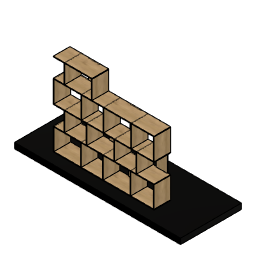
shelf v11 (Autodesk Fusion 360 design; units mm, degrees)
Autodesk Fusion 360 part; units mm, degrees
note: some values were not read from the file. Chosen so that the rebuilt part matches the saved one: which bodies a step acts on.
sketch "スケッチ1" plane through (0, 0, 0) normal (0, 1, 0) x (1, 0, 0)
  line L0 (0, 0) -> (1820, 0)
  line L1 (1820, 0) -> (1820, -300)
  line L2 (1820, -300) -> (0, -300)
  line L3 (0, -300) -> (0, 0)
  dimension "d1" = 1820
  dimension "d2" = 300
  constraint horizontal L0
  constraint vertical L1
  constraint horizontal L2
  constraint vertical L3
  constraint coincident L0.start L3.end
  measures "d1" distance of L0.start L0.end
  measures "d2" distance of L0.start L2.end
extrude "押し出し1" add sketch "スケッチ1" along normal blind 12 makes body 1
sketch "スケッチ2" plane through (0, 12, 0) normal (0, 1, 0) x (-1, 0, 0)
  line L0 (0, 300) -> (-1820, 300)
  line L1 (-1820, 300) -> (-1820, 0)
  line L2 (-1820, 0) -> (0, 0)
  line L3 (0, 0) -> (0, 300)
  line L4 (0, 0) -> (-12, 0)
  line L5 (-12, 0) -> (-12, 300)
  line L6 (-12, 300) -> (0, 300)
  line L7 (0, 300) -> (0, 0)
  line L8 (-12, 0) -> (-494, 0)
  line L9 (-494, 0) -> (-494, 300)
  line L10 (-494, 300) -> (-12, 300)
  line L11 (-12, 300) -> (-12, 0)
  line L12 (-494, 0) -> (-506, 0)
  line L13 (-506, 0) -> (-506, 300)
  line L14 (-506, 300) -> (-494, 300)
  line L15 (-494, 300) -> (-494, 0)
  line L16 (-506, 0) -> (-890, 0)
  line L17 (-890, 0) -> (-890, 300)
  line L18 (-890, 300) -> (-506, 300)
  line L19 (-506, 300) -> (-506, 0)
  line L20 (-890, 0) -> (-902, 0)
  line L21 (-902, 0) -> (-902, 300)
  line L22 (-902, 300) -> (-890, 300)
  line L23 (-890, 300) -> (-890, 0)
  line L24 (-902, 0) -> (-1290, 0)
  line L25 (-1290, 0) -> (-1290, 300)
  line L26 (-1290, 300) -> (-902, 300)
  line L27 (-902, 300) -> (-902, 0)
  dimension "d5" = 12
  dimension "d6" = 482
  dimension "d7" = 12
  dimension "d8" = 384
  dimension "d9" = 300
  dimension "d10" = 12
  dimension "d11" = 388
  constraint horizontal L4
  constraint vertical L5
  constraint horizontal L6
  constraint vertical L7
  constraint coincident L2.end L3.start
  constraint horizontal L8
  constraint vertical L9
  constraint horizontal L10
  constraint vertical L11
  constraint horizontal L12
  constraint vertical L13
  constraint horizontal L14
  constraint vertical L15
  constraint horizontal L16
  constraint vertical L17
  constraint horizontal L18
  constraint vertical L19
  constraint horizontal L20
  constraint vertical L21
  constraint horizontal L22
  constraint vertical L23
  constraint horizontal L24
  constraint vertical L25
  constraint horizontal L26
  constraint vertical L27
  measures "d5" distance of L2.end L4.end
  measures "d6" distance of L4.end L8.end
  measures "d7" distance of L8.end L12.end
  measures "d8" distance of L12.end L16.end
  measures "d9" distance of L12.end L13.end
  measures "d10" distance of L16.end L20.end
  measures "d11" distance of L20.end L24.end
sketch "スケッチ3" plane through (0, 12, 0) normal (0, 1, 0) x (-1, 0, 0)
  line L0 (-900, 0) -> (-1388, 0)
  line L1 (-1388, 0) -> (-1388, 300)
  line L2 (-1388, 300) -> (-900, 300)
  line L3 (-900, 300) -> (-900, 0)
  line L4 (-1820, 0) -> (-1808, 0)
  line L5 (-1808, 0) -> (-1808, 300)
  line L6 (-1808, 300) -> (-1820, 300)
  line L7 (-1820, 300) -> (-1820, 0)
  line L8 (-1388, 0) -> (-1808, 0)
  line L9 (-1808, 0) -> (-1808, 300)
  line L10 (-1808, 300) -> (-1388, 300)
  line L11 (-1388, 300) -> (-1388, 0)
  line L12 (-1388, 0) -> (-1400, 0)
  line L13 (-1400, 0) -> (-1400, 300)
  line L14 (-1400, 300) -> (-1388, 300)
  line L15 (-1388, 300) -> (-1388, 0)
  dimension "d12" = 488
  dimension "d13" = 12
  dimension "d14" = 300
  dimension "d15" = 12
  constraint horizontal L0
  constraint vertical L1
  constraint horizontal L2
  constraint vertical L3
  constraint horizontal L4
  constraint vertical L5
  constraint horizontal L6
  constraint vertical L7
  constraint horizontal L8
  constraint vertical L9
  constraint horizontal L10
  constraint vertical L11
  constraint horizontal L12
  constraint vertical L13
  constraint horizontal L14
  constraint vertical L15
  measures "d12" distance of L0.start L0.end
  measures "d13" distance of L4.start L4.end
  measures "d14" distance of L0.end L1.end
  measures "d15" distance of L0.end L12.end
extrude "押し出し2" add sketch "スケッチ3" sketch "スケッチ2" along normal blind 382 separate body contours L1 L8 L10 L11 L12 L13 L14 L15 | L4 L5 L6 L7 L9 of sketch 2 contours L0 L2 L3 L4 L5 L6 L7 L11 | L0 L2 L9 L12 L13 L14 L15 L19 | L0 L2 L17 L20 L21 L22 L23 L27 makes body 2 at (0, 266.6667, 100) makes body 3 at (1820, 266.6667, 200) makes body 4 at (1400, 266.6667, 100) makes body 5 at (494, 266.6667, 100) makes body 6 at (890, 266.6667, 100)
sketch "スケッチ7" plane through (0, 394, 0) normal (0, 1, 0) x (-1, 0, 0)
  line L0 (0, 300) -> (-12, 300)
  line L1 (-12, 300) -> (-12, 0)
  line L2 (-12, 0) -> (0, 0)
  line L3 (0, 0) -> (0, 300)
  line L4 (0, 0) -> (-1820, 0)
  line L5 (-1820, 0) -> (-1820, 300)
  line L6 (-1820, 300) -> (0, 300)
  line L7 (0, 300) -> (0, 0)
  constraint horizontal L4
  constraint vertical L5
  constraint horizontal L6
  constraint vertical L7
  constraint coincident L2.end L3.start
extrude "押し出し4" add sketch "スケッチ7" along normal blind 12 separate body contours L1 L4 L5 L6 makes body 7
extrude "押し出し5" add 1 faces at (12, 398, 200) along direction (-1, 0, 0) blind 12 on bodies 7 bodies 7 2
split "分割1" by plane through (0, 394, 0) normal (0, -1, 0) bodies 7 makes body 8 at (0, 139.3333, 200)
sketch "スケッチ8" plane through (0, 406, 0) normal (0, 1, 0) x (-1, 0, 0)
  line L0 (-1820, 300) -> (-1820, 0)
  line L1 (-1820, 0) -> (0, 0)
  line L2 (0, 0) -> (0, 300)
  line L3 (0, 300) -> (-1820, 300)
  line L4 (0, 0) -> (-194, 0)
  line L5 (-194, 0) -> (-194, 300)
  line L6 (-194, 300) -> (0, 300)
  line L7 (0, 300) -> (0, 0)
  line L8 (-194, 0) -> (-206, 0)
  line L9 (-206, 0) -> (-206, 300)
  line L10 (-206, 300) -> (-194, 300)
  line L11 (-194, 300) -> (-194, 0)
  line L12 (-206, 0) -> (-594, 0)
  line L13 (-594, 0) -> (-594, 300)
  line L14 (-594, 300) -> (-206, 300)
  line L15 (-206, 300) -> (-206, 0)
  line L16 (-594, 0) -> (-606, 0)
  line L17 (-606, 0) -> (-606, 300)
  line L18 (-606, 300) -> (-594, 300)
  line L19 (-594, 300) -> (-594, 0)
  line L20 (-606, 0) -> (-1094, 0)
  line L21 (-1094, 0) -> (-1094, 300)
  line L22 (-1094, 300) -> (-606, 300)
  line L23 (-606, 300) -> (-606, 0)
  line L24 (-1094, 0) -> (-1106, 0)
  line L25 (-1106, 0) -> (-1106, 300)
  line L26 (-1106, 300) -> (-1094, 300)
  line L27 (-1094, 300) -> (-1094, 0)
  line L28 (-1106, 0) -> (-1494, 0)
  line L29 (-1494, 0) -> (-1494, 300)
  line L30 (-1494, 300) -> (-1106, 300)
  line L31 (-1106, 300) -> (-1106, 0)
  line L32 (-1494, 0) -> (-1506, 0)
  line L33 (-1506, 0) -> (-1506, 300)
  line L34 (-1506, 300) -> (-1494, 300)
  line L35 (-1494, 300) -> (-1494, 0)
  dimension "d34" = 194
  dimension "d35" = 12
  dimension "d36" = 388
  dimension "d37" = 300
  dimension "d38" = 12
  dimension "d39" = 488
  dimension "d40" = 12
  dimension "d41" = 388
  dimension "d42" = 300
  dimension "d43" = 12
  constraint horizontal L4
  constraint vertical L5
  constraint horizontal L6
  constraint vertical L7
  constraint coincident L1.end L2.start
  constraint horizontal L8
  constraint vertical L9
  constraint horizontal L10
  constraint vertical L11
  constraint horizontal L12
  constraint vertical L13
  constraint horizontal L14
  constraint vertical L15
  constraint horizontal L16
  constraint vertical L17
  constraint horizontal L18
  constraint vertical L19
  constraint horizontal L20
  constraint vertical L21
  constraint horizontal L22
  constraint vertical L23
  constraint horizontal L24
  constraint vertical L25
  constraint horizontal L26
  constraint vertical L27
  constraint horizontal L28
  constraint vertical L29
  constraint horizontal L30
  constraint vertical L31
  constraint horizontal L32
  constraint vertical L33
  constraint horizontal L34
  constraint vertical L35
  measures "d34" distance of L1.end L4.end
  measures "d35" distance of L4.end L8.end
  measures "d36" distance of L8.end L12.end
  measures "d37" distance of L8.end L9.end
  measures "d38" distance of L12.end L16.end
  measures "d39" distance of L16.end L20.end
  measures "d40" distance of L20.end L24.end
  measures "d41" distance of L24.end L28.end
  measures "d42" distance of L24.end L25.end
  measures "d43" distance of L28.end L32.end
extrude "押し出し6" add sketch "スケッチ8" along normal blind 338 separate body contours L1 L3 L29 L32 L33 L34 L35 | L1 L3 L21 L24 L25 L26 L27 L31 | L1 L3 L13 L16 L17 L18 L19 L23 | L1 L3 L5 L8 L9 L10 L11 L15 makes body 9 at (594, 631.3333, 100) makes body 10 at (1094, 631.3333, 100) makes body 11 at (194, 631.3333, 100) makes body 12 at (1494, 631.3333, 100)
sketch "スケッチ9" plane through (0, 744, 0) normal (0, 1, 0) x (-1, 0, 0)
  line L0 (-194, 300) -> (-206, 300)
  line L1 (-206, 300) -> (-206, 0)
  line L2 (-206, 0) -> (-194, 0)
  line L3 (-194, 0) -> (-194, 300)
  line L4 (0, 0) -> (-1820, 0)
  line L5 (-1820, 0) -> (-1820, 300)
  line L6 (-1820, 300) -> (0, 300)
  line L7 (0, 300) -> (0, 0)
  constraint horizontal L4
  constraint vertical L5
  constraint horizontal L6
  constraint vertical L7
  constraint coincident L4.start L7.end
extrude "押し出し7" add sketch "スケッチ9" along normal blind 12 separate body contours L1 L4 L5 L6 makes body 13
move_face "面をオフセット1" offset 200 1 faces at (206, 748, 200) on bodies 13
extrude "押し出し8" add 1 faces at (6, 748, 200) along direction (-1, 0, 0) blind 6 on bodies 13 bodies 13
sketch "スケッチ10" plane through (0, 756, 0) normal (0, 1, 0) x (-1, 0, 0)
  line L0 (-1820, 300) -> (-1820, 0)
  line L1 (-1820, 0) -> (0, 0)
  line L2 (0, 0) -> (0, 300)
  line L3 (0, 300) -> (-1820, 300)
  line L4 (0, 0) -> (-12, 0)
  line L5 (-12, 0) -> (-12, 300)
  line L6 (-12, 300) -> (0, 300)
  line L7 (0, 300) -> (0, 0)
  line L8 (-12, 0) -> (-500, 0)
  line L9 (-500, 0) -> (-500, 300)
  line L10 (-500, 300) -> (-12, 300)
  line L11 (-12, 300) -> (-12, 0)
  line L12 (-500, 0) -> (-512, 0)
  line L13 (-512, 0) -> (-512, 300)
  line L14 (-512, 300) -> (-500, 300)
  line L15 (-500, 300) -> (-500, 0)
  line L16 (-512, 0) -> (-900, 0)
  line L17 (-900, 0) -> (-900, 300)
  line L18 (-900, 300) -> (-512, 300)
  line L19 (-512, 300) -> (-512, 0)
  line L20 (-900, 0) -> (-912, 0)
  line L21 (-912, 0) -> (-912, 300)
  line L22 (-912, 300) -> (-900, 300)
  line L23 (-900, 300) -> (-900, 0)
  line L24 (-912, 0) -> (-1400, 0)
  line L25 (-1400, 0) -> (-1400, 300)
  line L26 (-1400, 300) -> (-912, 300)
  line L27 (-912, 300) -> (-912, 0)
  line L28 (-1400, 0) -> (-1412, 0)
  line L29 (-1412, 0) -> (-1412, 300)
  line L30 (-1412, 300) -> (-1400, 300)
  line L31 (-1400, 300) -> (-1400, 0)
  line L32 (-1412, 0) -> (-1808, 0)
  line L33 (-1808, 0) -> (-1808, 300)
  line L34 (-1808, 300) -> (-1412, 300)
  line L35 (-1412, 300) -> (-1412, 0)
  dimension "d51" = 12
  dimension "d52" = 488
  dimension "d53" = 12
  dimension "d54" = 388
  dimension "d55" = 12
  dimension "d56" = 488
  dimension "d57" = 12
  dimension "d58" = 396
  dimension "d59" = 300
  constraint horizontal L4
  constraint vertical L5
  constraint horizontal L6
  constraint vertical L7
  constraint coincident L1.end L2.start
  constraint horizontal L8
  constraint vertical L9
  constraint horizontal L10
  constraint vertical L11
  constraint horizontal L12
  constraint vertical L13
  constraint horizontal L14
  constraint vertical L15
  constraint horizontal L16
  constraint vertical L17
  constraint horizontal L18
  constraint vertical L19
  constraint horizontal L20
  constraint vertical L21
  constraint horizontal L22
  constraint vertical L23
  constraint horizontal L24
  constraint vertical L25
  constraint horizontal L26
  constraint vertical L27
  constraint horizontal L28
  constraint vertical L29
  constraint horizontal L30
  constraint vertical L31
  constraint horizontal L32
  constraint vertical L33
  constraint horizontal L34
  constraint vertical L35
  measures "d51" distance of L1.end L4.end
  measures "d52" distance of L4.end L8.end
  measures "d53" distance of L8.end L12.end
  measures "d54" distance of L12.end L16.end
  measures "d55" distance of L16.end L20.end
  measures "d56" distance of L20.end L24.end
  measures "d57" distance of L24.end L28.end
  measures "d58" distance of L28.end L32.end
  measures "d59" distance of L28.end L29.end
extrude "押し出し9" add sketch "スケッチ10" along normal blind 388 separate body contours L0 L1 L3 L33 | L1 L3 L25 L28 L29 L30 L31 L35 | L1 L3 L17 L20 L21 L22 L23 L27 | L1 L3 L9 L12 L13 L14 L15 L19 | L1 L2 L3 L4 L5 L6 L7 L11 makes body 14 at (900, 1014.6667, 100) makes body 15 at (1400, 1014.6667, 100) makes body 16 at (500, 1014.6667, 100) makes body 17 at (1820, 1014.6667, 200) makes body 18 at (0, 1014.6667, 100)
sketch "スケッチ11" plane through (0, 1144, 0) normal (0, 1, 0) x (-1, 0, 0)
  line L0 (0, 300) -> (-12, 300)
  line L1 (-12, 300) -> (-12, 0)
  line L2 (-12, 0) -> (0, 0)
  line L3 (0, 0) -> (0, 300)
  line L4 (0, 0) -> (-1820, 0)
  line L5 (-1820, 0) -> (-1820, 300)
  line L6 (-1820, 300) -> (0, 300)
  line L7 (0, 300) -> (0, 0)
  constraint horizontal L4
  constraint vertical L5
  constraint horizontal L6
  constraint vertical L7
  constraint coincident L2.end L3.start
extrude "押し出し10" add sketch "スケッチ11" along normal blind 12 separate body makes body 19
sketch "スケッチ12" plane through (0, 1156, 0) normal (0, 1, 0) x (-1, 0, 0)
  line L0 (0, 300) -> (-1820, 300)
  line L1 (-1820, 300) -> (-1820, 0)
  line L2 (-1820, 0) -> (0, 0)
  line L3 (0, 0) -> (0, 300)
  line L4 (0, 0) -> (-12, 0)
  line L5 (-12, 0) -> (-12, 300)
  line L6 (-12, 300) -> (0, 300)
  line L7 (0, 300) -> (0, 0)
  line L8 (-12, 0) -> (-194, 0)
  line L9 (-194, 0) -> (-194, 300)
  line L10 (-194, 300) -> (-12, 300)
  line L11 (-12, 300) -> (-12, 0)
  line L12 (-194, 0) -> (-206, 0)
  line L13 (-206, 0) -> (-206, 300)
  line L14 (-206, 300) -> (-194, 300)
  line L15 (-194, 300) -> (-194, 0)
  line L16 (-206, 0) -> (-688, 0)
  line L17 (-688, 0) -> (-688, 300)
  line L18 (-688, 300) -> (-206, 300)
  line L19 (-206, 300) -> (-206, 0)
  line L20 (-688, 0) -> (-700, 0)
  line L21 (-700, 0) -> (-700, 300)
  line L22 (-700, 300) -> (-688, 300)
  line L23 (-688, 300) -> (-688, 0)
  dimension "d64" = 12
  dimension "d65" = 182
  dimension "d66" = 12
  dimension "d67" = 482
  dimension "d68" = 300
  dimension "d69" = 12
  constraint horizontal L4
  constraint vertical L5
  constraint horizontal L6
  constraint vertical L7
  constraint coincident L2.end L3.start
  constraint horizontal L8
  constraint vertical L9
  constraint horizontal L10
  constraint vertical L11
  constraint horizontal L12
  constraint vertical L13
  constraint horizontal L14
  constraint vertical L15
  constraint horizontal L16
  constraint vertical L17
  constraint horizontal L18
  constraint vertical L19
  constraint horizontal L20
  constraint vertical L21
  constraint horizontal L22
  constraint vertical L23
  measures "d64" distance of L2.end L4.end
  measures "d65" distance of L4.end L8.end
  measures "d66" distance of L8.end L12.end
  measures "d67" distance of L12.end L16.end
  measures "d68" distance of L12.end L13.end
  measures "d69" distance of L16.end L20.end
sketch "スケッチ13" plane through (0, 1488, 0) normal (0, 1, 0) x (-1, 0, 0)
  line L0 (0, 300) -> (-12, 300)
  line L1 (-12, 300) -> (-12, 0)
  line L2 (-12, 0) -> (0, 0)
  line L3 (0, 0) -> (0, 300)
  line L4 (0, 0) -> (-700, 0)
  line L5 (-700, 0) -> (-700, 300)
  line L6 (-700, 300) -> (0, 300)
  line L7 (0, 300) -> (0, 0)
  constraint horizontal L4
  constraint vertical L5
  constraint horizontal L6
  constraint vertical L7
  constraint coincident L2.end L3.start
extrude "押し出し12" add sketch "スケッチ13" along normal blind 12 separate body makes body 20
sketch "スケッチ14" plane through (0, 0, 0) normal (0, 0, -1) x (-1, 0, 0)
  line L0 (-1820, 394) -> (0, 394)
  line L1 (0, 394) -> (0, 406)
  line L2 (0, 406) -> (-1820, 406)
  line L3 (-1820, 406) -> (-1820, 394)
  line L4 (-402.3819, 406) -> (-222.3819, 406)
  line L5 (-222.3819, 406) -> (-222.3819, 0)
  line L6 (-222.3819, 0) -> (-402.3819, 0)
  line L7 (-402.3819, 0) -> (-402.3819, 406)
  dimension "d74" = 180
  constraint horizontal L4
  constraint vertical L5
  constraint horizontal L6
  constraint vertical L7
  constraint coincident L2 L4.start
  measures "d74" distance of L4.start L4.end
extrude "押し出し13" add sketch "スケッチ14" along normal blind 12 separate body contours L0 L2 L4 L5 L7 | L0 L5 L6 L7 makes body 21
sketch "スケッチ15" plane through (0, 0, 0) normal (0, 0, -1) x (-1, 0, 0)
  line L0 (-1820, 744) -> (0, 744)
  line L1 (0, 744) -> (0, 756)
  line L2 (0, 756) -> (-1820, 756)
  line L3 (-1820, 756) -> (-1820, 744)
  line L4 (-400.5318, 1143.8543) -> (-220.5318, 1143.8543)
  line L5 (-220.5318, 1143.8543) -> (-220.5318, 755.8543)
  line L6 (-220.5318, 755.8543) -> (-400.5318, 755.8543)
  line L7 (-400.5318, 755.8543) -> (-400.5318, 1143.8543)
  dimension "d77" = 180
  dimension "d78" = 388
  constraint horizontal L4
  constraint vertical L5
  constraint horizontal L6
  constraint vertical L7
  measures "d77" distance of L4.start L4.end
  measures "d78" distance of L4.start L6.end
extrude "押し出し14" add sketch "スケッチ15" along normal blind 12 separate body contours L2 L4 L5 L7 makes body 22
move_body "移動5" bodies 22 to x (1, 0, 0) y (0, 1, 0) z (0, 0, 1) at (0, 0, 12)
sketch "スケッチ16" plane through (0, 0, 0) normal (0, 0, -1) x (-1, 0, 0)
  line L0 (-700, 1488) -> (0, 1488)
  line L1 (0, 1488) -> (0, 1500)
  line L2 (0, 1500) -> (-700, 1500)
  line L3 (-700, 1500) -> (-700, 1488)
  line L4 (-548.7632, 1488) -> (-398.7632, 1488)
  line L5 (-398.7632, 1488) -> (-398.7632, 1156)
  line L6 (-398.7632, 1156) -> (-548.7632, 1156)
  line L7 (-548.7632, 1156) -> (-548.7632, 1488)
  dimension "d81" = 150
  dimension "d82" = 332
  constraint horizontal L4
  constraint vertical L5
  constraint horizontal L6
  constraint vertical L7
  constraint coincident L0 L4.start
  measures "d81" distance of L4.start L4.end
  measures "d82" distance of L4.start L6.end
extrude "押し出し15" add sketch "スケッチ16" against normal blind 12 separate body contours L0 L4 L5 L6 L7 makes body 23
move_body "移動6" bodies 23 to x (1, 0, 0) y (0, 1, 0) z (0, 0, 1) at (0, 0, -100)
extrude "押し出し16" add 1 faces at (398.7632, 1377.3333, -96) along direction (-1, 0, 0) blind 50 on bodies 23 bodies 23
move_body "移動7" bodies 23 to x (1, 0, 0) y (0, 1, 0) z (0, 0, 1) at (0, 0, 100)
sketch "スケッチ17" plane through (0, 0, 0) normal (0, 0, -1) x (-1, 0, 0)
  line L0 (-1820, 744) -> (0, 744)
  line L1 (0, 744) -> (0, 756)
  line L2 (0, 756) -> (-1820, 756)
  line L3 (-1820, 756) -> (-1820, 744)
  line L4 (-923.4026, 744) -> (-723.4026, 744)
  line L5 (-723.4026, 744) -> (-723.4026, 406)
  line L6 (-723.4026, 406) -> (-923.4026, 406)
  line L7 (-923.4026, 406) -> (-923.4026, 744)
  dimension "d87" = 200
  dimension "d88" = 338
  constraint horizontal L4
  constraint vertical L5
  constraint horizontal L6
  constraint vertical L7
  constraint coincident L0 L4.start
  measures "d87" distance of L4.start L4.end
  measures "d88" distance of L4.start L6.end
sketch "スケッチ18" plane through (0, 0, 0) normal (0, 0, -1) x (-1, 0, 0)
  line L0 (-1820, 1144) -> (0, 1144)
  line L1 (0, 1144) -> (0, 1156)
  line L2 (0, 1156) -> (-1820, 1156)
  line L3 (-1820, 1156) -> (-1820, 1144)
  line L4 (-1299.0932, 1144) -> (-1099.0932, 1144)
  line L5 (-1099.0932, 1144) -> (-1099.0932, 756)
  line L6 (-1099.0932, 756) -> (-1299.0932, 756)
  line L7 (-1299.0932, 756) -> (-1299.0932, 1144)
  dimension "d89" = 200
  dimension "d90" = 388
  constraint horizontal L4
  constraint vertical L5
  constraint horizontal L6
  constraint vertical L7
  constraint coincident L0 L4.start
  measures "d89" distance of L4.start L4.end
  measures "d90" distance of L4.start L6.end
sketch "スケッチ19" plane through (0, 0, 0) normal (0, 0, -1) x (-1, 0, 0)
  line L0 (-1820, 394) -> (0, 394)
  line L1 (0, 394) -> (0, 406)
  line L2 (0, 406) -> (-1820, 406)
  line L3 (-1820, 406) -> (-1820, 394)
  line L4 (-1271.1858, 394) -> (-1071.1858, 394)
  line L5 (-1071.1858, 394) -> (-1071.1858, 12)
  line L6 (-1071.1858, 12) -> (-1271.1858, 12)
  line L7 (-1271.1858, 12) -> (-1271.1858, 394)
  dimension "d91" = 200
  dimension "d92" = 382
  constraint horizontal L4
  constraint vertical L5
  constraint horizontal L6
  constraint vertical L7
  constraint coincident L0 L4.start
  measures "d91" distance of L4.start L4.end
  measures "d92" distance of L4.start L6.end
extrude "押し出し17" cut 1 faces at (282.3819, 0, -8) along direction (0, 1, 0) blind 24 on bodies 21 bodies 21
move_body "移動8" bodies 21 to x (1, 0, 0) y (0, 1, 0) z (0, 0, 1) at (0, -12, 12)
extrude "押し出し18" add sketch "スケッチ17" sketch "スケッチ18" sketch "スケッチ19" against normal blind 12 separate body contours L0 L4 L5 L6 L7 of sketch 2 contours L0 L4 L5 L6 L7 of sketch 3 contours L0 L4 L5 L6 L7 makes body 24 at (1165.7599, 885.3333, 0) makes body 25 at (856.7359, 631.3333, 0) makes body 26 at (1204.5191, 266.6667, 0)
sketch "スケッチ20" plane through (0, 1488, 0) normal (0, -1, 0) x (1, 0, 0)
  line L0 (700, 300) -> (0, 300)
  line L1 (0, 300) -> (0, 0)
  line L2 (0, 0) -> (700, 0)
  line L3 (700, 0) -> (700, 300)
  line L4 (700, 300) -> (688, 300)
  line L5 (688, 300) -> (688, 0)
  line L6 (688, 0) -> (700, 0)
  line L7 (700, 0) -> (700, 300)
  line L8 (688, 300) -> (206, 300)
  line L9 (206, 300) -> (206, 0)
  line L10 (206, 0) -> (688, 0)
  line L11 (688, 0) -> (688, 300)
  line L12 (206, 300) -> (194, 300)
  line L13 (194, 300) -> (194, 0)
  line L14 (194, 0) -> (206, 0)
  line L15 (206, 0) -> (206, 300)
  dimension "d97" = 12
  dimension "d98" = 482
  dimension "d99" = 12
  constraint horizontal L4
  constraint vertical L5
  constraint horizontal L6
  constraint vertical L7
  constraint coincident L0.start L3.end
  constraint horizontal L8
  constraint vertical L9
  constraint horizontal L10
  constraint vertical L11
  constraint horizontal L12
  constraint vertical L13
  constraint horizontal L14
  constraint vertical L15
  measures "d97" distance of L0.start L4.end
  measures "d98" distance of L4.end L8.end
  measures "d99" distance of L8.end L12.end
extrude "押し出し19" add sketch "スケッチ20" along normal blind 332 separate body contours L0 L2 L3 L4 L5 L6 L7 L11 | L0 L2 L9 L12 L13 L14 L15 makes body 27 at (700, 1377.3333, 100) makes body 28 at (206, 1377.3333, 200)
sketch "スケッチ21" plane through (0, 0, 0) normal (0, 1, 0) x (1, 0, 0)
  line L0 (-500, -500) -> (2500, -500)
  line L1 (2500, -500) -> (2500, 600)
  line L2 (2500, 600) -> (-500, 600)
  line L3 (-500, 600) -> (-500, -500)
  constraint horizontal L0
  constraint vertical L1
  constraint horizontal L2
  constraint vertical L3
extrude "押し出し20" add sketch "スケッチ21" against normal blind 100 separate body makes body 29
copy_body "ボディのコピーと貼り付け5" bodies 25 makes body 30
move_body "移動9" bodies 30 to x (1, 0, 0) y (0, 1, 0) z (0, 0, 1) at (850, 0, 0)
sketch "スケッチ4" plane through (0, 394, 0) normal (0, 1, 0) x (-1, 0, 0)
  line L0 (0, 0) -> (-1820, 0)
  line L1 (-1820, 0) -> (-1820, 300)
  line L2 (-1820, 300) -> (0, 300)
  line L3 (0, 300) -> (0, 0)
  line L4 (0, 0) -> (-140, 0)
  line L5 (-140, 0) -> (-140, 300)
  line L6 (-140, 300) -> (0, 300)
  line L7 (0, 300) -> (0, 0)
  line L8 (-140, 0) -> (-152, 0)
  line L9 (-152, 0) -> (-152, 300)
  line L10 (-152, 300) -> (-140, 300)
  line L11 (-140, 300) -> (-140, 0)
  line L12 (-152, 0) -> (-540, 0)
  line L13 (-540, 0) -> (-540, 300)
  line L14 (-540, 300) -> (-152, 300)
  line L15 (-152, 300) -> (-152, 0)
  line L16 (-540, 0) -> (-552, 0)
  line L17 (-552, 0) -> (-552, 300)
  line L18 (-552, 300) -> (-540, 300)
  line L19 (-540, 300) -> (-540, 0)
  line L20 (-552, 0) -> (-1040, 0)
  line L21 (-1040, 0) -> (-1040, 300)
  line L22 (-1040, 300) -> (-552, 300)
  line L23 (-552, 300) -> (-552, 0)
  line L24 (-1040, 0) -> (-1052, 0)
  line L25 (-1052, 0) -> (-1052, 300)
  line L26 (-1052, 300) -> (-1040, 300)
  line L27 (-1040, 300) -> (-1040, 0)
  line L28 (-890, 300) -> (-902, 300)
  line L29 (-902, 300) -> (-902, 0)
  line L30 (-902, 0) -> (-890, 0)
  line L31 (-890, 0) -> (-890, 300)
  line L32 (-494, 300) -> (-506, 300)
  line L33 (-506, 300) -> (-506, 0)
  line L34 (-506, 0) -> (-494, 0)
  line L35 (-494, 0) -> (-494, 300)
  line L36 (-1388, 300) -> (-1400, 300)
  line L37 (-1400, 300) -> (-1400, 0)
  line L38 (-1400, 0) -> (-1388, 0)
  line L39 (-1388, 0) -> (-1388, 300)
  line L40 (-1808, 0) -> (-1808, 300)
  line L41 (-1808, 300) -> (-1820, 300)
  line L42 (-1820, 300) -> (-1820, 0)
  line L43 (-1820, 0) -> (-1808, 0)
  dimension "d18" = 140
  dimension "d19" = 12
  dimension "d20" = 300
  dimension "d21" = 388
  dimension "d22" = 12
  dimension "d23" = 488
  dimension "d24" = 300
  dimension "d25" = 12
  constraint horizontal L0
  constraint vertical L1
  constraint horizontal L2
  constraint vertical L3
  constraint horizontal L4
  constraint vertical L5
  constraint horizontal L6
  constraint vertical L7
  constraint horizontal L8
  constraint vertical L9
  constraint horizontal L10
  constraint vertical L11
  constraint horizontal L12
  constraint vertical L13
  constraint horizontal L14
  constraint vertical L15
  constraint horizontal L16
  constraint vertical L17
  constraint horizontal L18
  constraint vertical L19
  constraint horizontal L20
  constraint vertical L21
  constraint horizontal L22
  constraint vertical L23
  constraint horizontal L24
  constraint vertical L25
  constraint horizontal L26
  constraint vertical L27
  measures "d18" distance of L0.start L4.end
  measures "d19" distance of L4.end L8.end
  measures "d20" distance of L4.end L5.end
  measures "d21" distance of L8.end L12.end
  measures "d22" distance of L12.end L16.end
  measures "d23" distance of L16.end L20.end
  measures "d24" distance of L16.end L17.end
  measures "d25" distance of L20.end L24.end
sketch "スケッチ5" plane through (0, 394, 0) normal (0, 1, 0) x (-1, 0, 0)
  line L0 (-1050, 0) -> (-1438, 0)
  line L1 (-1438, 0) -> (-1438, 300)
  line L2 (-1438, 300) -> (-1050, 300)
  line L3 (-1050, 300) -> (-1050, 0)
  line L4 (-1438, 0) -> (-1450, 0)
  line L5 (-1450, 0) -> (-1450, 300)
  line L6 (-1450, 300) -> (-1438, 300)
  line L7 (-1438, 300) -> (-1438, 0)
  dimension "d26" = 388
  dimension "d27" = 12
  constraint horizontal L0
  constraint vertical L1
  constraint horizontal L2
  constraint vertical L3
  constraint horizontal L4
  constraint vertical L5
  constraint horizontal L6
  constraint vertical L7
  measures "d26" distance of L0.start L0.end
  measures "d27" distance of L0.end L4.end
extrude "押し出し3" [suppressed]
sketch "スケッチ6" plane through (0, 394, 0) normal (0, 1, 0) x (-1, 0, 0)
